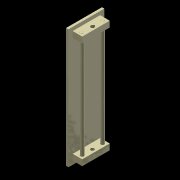
# Autodesk Inventor part: Bearing2
Saved by Autodesk Inventor 2020 (Build 240168000, 168)
## iProperties
Created: 2019-08-02
Part Number: Bearing2
Document SubType Name: Modeling
Designer: Administrator
Density: 1 g/cm^3
Mass: 8.86804 g
Surface Area: 93.5607 cm^2
Volume: 8.86804 cm^3
Material: 一般
Appearance: 尼龍 6
Author: Administrator
Autodesk Inventor part; units mm, degrees
ref_plane "YZ Plane" through (0, 0, 0) normal (1, 0, 0) x (0, 1, 0)
ref_plane "XZ Plane" through (0, 0, 0) normal (0, 1, 0) x (-1, 0, 0)
sketch "Sketch1" plane through (0, 0, 0) normal (0, 0, 1) x (1, 0, 0)
  circle A0 centre (0, 0) radius 1.5
  line L0 (3, 3) -> (3, -3)
  line L1 (3, -3) -> (-3, -3)
  line L2 (-3, -3) -> (-3, 3)
  line L3 (-3, 3) -> (3, 3)
  dimension "d0" = 3
  dimension "d1" = 6
  constraints: 8 end point, 1 centre point, 1 coincident, 10 other
  measures "d0" diameter of A0
  measures "d1" distance of L2.end L0.start
extrude "Extrusion1" add sketch "Sketch1" along normal blind 5
sketch "Sketch13" plane through (0, 0, 0) normal (0, 0, -1) x (-1, 0, 0)
  circle A0 centre (0, 0) radius 1.5 projected
  line L0 (3, 3) -> (-3, 3) projected
  line L1 (0, 0) -> (0, 1.5)
  circle A1 centre (0, 1.5) radius 0.5
  dimension "d63" = 1
  constraints: 2 end point, 1 centre point, 1 coincident, 1 perpendicular, 1 vertical alignment, 1 other
  measures "d63" diameter of A1
extrude "Extrusion11" cut sketch "Sketch13" against normal blind 2 contours A1 L1 A0 | A0 A1 | A0 L1 A1 picked at (-0.1081, 1.6551)
thread "Thread2" size "M1x0.25" class "6H" standard "ANSI Metric M Profile" full length
ref_plane "Work Plane3" through (0, 0, 47) normal (0, 0, 1) x (1, 0, 0)
sketch "Sketch15" plane through (0, 0, 0) normal (0, 0, -1) x (-1, 0, 0)
  line L0 (-3, 3) -> (-3, -3) projected
  line L1 (3, -3) -> (3, 3) projected
  line L2 (3, 3) -> (-3, 3) projected
  arc A0 (-0.493, 1.4167) -> (0.493, 1.4167) centre (0, 0) ccw projected
  line L3 (0, 0) -> (0, 3) construction
  line L4 (0, 0) -> (0, 8.5) construction
  circle A1 centre (0, 8.5) radius 1.5
  line L5 (-3, 3) -> (3, 3)
  line L6 (3, 3) -> (3, 11.5)
  line L7 (3, 11.5) -> (-3, 11.5)
  line L8 (-3, 11.5) -> (-3, 3)
  line L9 (-3, 0) -> (3, 0) construction
  line L10 (3, -3) -> (-3, -3)
  circle A2 centre (0, -8.5) radius 1.5
  line L11 (-3, -3) -> (3, -3)
  line L12 (3, -3) -> (3, -11.5)
  line L13 (3, -11.5) -> (-3, -11.5)
  line L14 (-3, -11.5) -> (-3, -3)
  point P0 (0, -3)
  dimension "d76" = 3
  dimension "d77" = 8.5
  dimension "d78" = 3
  constraints: 24 end point, 7 symmetric about line, 3 midpoint, 2 centre point, 2 coincident, 2 parallel, 1 horizontal, 1 perpendicular, 1 point on line, 1 other
  measures "d76" diameter of A1
  measures "d77" distance of L3.start L4.end
  measures "d78" distance from line of L7 L4.end
extrude "Extrusion13" add sketch "Sketch15" against normal up to surface (5 mm away) contours L8 L7 L6 L2 | L10 L12 L13 L14
mirror "Mirror2" about plane through (0, 0, 47) normal (0, 0, 1) of "Extrusion1", "Extrusion11", "Extrusion13"
sketch "Sketch16" plane through (0, 0, 0) normal (0, 0, -1) x (-1, 0, 0)
  circle A0 centre (0, 8.5) radius 1.5 projected
  circle A1 centre (0, -8.5) radius 1.5 projected
  circle A2 centre (0, 8.5) radius 1.45
  circle A3 centre (0, -8.5) radius 1.45
  dimension "d81" = 0.05
  constraints: 2 centre point, 1 equal radius
  measures "d81" radial gap between concentric circles of A2 A0
extrude "Extrusion14" add sketch "Sketch16" against normal up to surface (94 mm away) contours A2 | A3
sketch "Sketch17" plane through (-3, -11.5, 5) normal (-1, 0, 0) x (0, 0, 1)
  line L0 (0, 0) -> (0, 23) projected
  line L1 (-5, 23) -> (0, 23) projected
  line L2 (-5, 0) -> (-5, 23) projected
  line L3 (-5, 0) -> (0, 0) projected
  line L4 (84, 0) -> (84, 23) projected
  line L5 (89, 0) -> (84, 0) projected
  line L6 (89, 0) -> (89, 23) projected
  line L7 (89, 23) -> (84, 23) projected
extrude "Extrusion15" add sketch "Sketch17" along normal blind 2
sketch "Sketch18" plane through (-5, -11.5, 5) normal (-1, 0, 0) x (0, 0, 1)
  line L0 (84, 23) -> (89, 23) projected
  line L1 (84, 0) -> (84, 23) projected
  line L2 (89, 0) -> (84, 0) projected
  line L3 (89, 23) -> (89, 0) projected
  line L4 (-8, 26.5) -> (92, 26.5)
  line L5 (92, 26.5) -> (92, -3.5)
  line L6 (92, -3.5) -> (-8, -3.5)
  line L7 (-8, -3.5) -> (-8, 26.5)
  line L8 (89, 23) -> (89, 26.5) construction
  line L9 (89, 0) -> (89, -3.5) construction
  line L10 (89, 0) -> (92, 0) construction
  line L11 (-5, 0) -> (-8, 0) construction
  dimension "d86" = 30
  dimension "d87" = 100
  constraints: 16 end point, 4 perpendicular, 4 point on line, 3 parallel, 2 collinear, 1 horizontal
  measures "d86" distance between parallel lines of L4 L6
  measures "d87" distance of L4.start L4.end
extrude "Extrusion16" add sketch "Sketch18" along normal blind 2 contours L0 L3 L2 L1 | L4 L5 L6 L7
